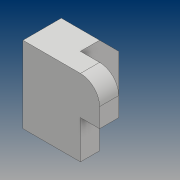
# Autodesk Inventor part: 47 (28785.398 mm^3)
Saved by Autodesk Inventor 2018 (Build 220112000, 112)
## iProperties
Created: 2020-09-18
Part Number: 47 (28785.398 mm^3)
Material: 一般
Document SubType Name: Modeling
Designer: 88697
Density: 1 g/cm^3
Appearance: 預設
Author: 88697
Autodesk Inventor part; units mm, degrees
ref_plane "YZ Plane" through (0, 0, 0) normal (1, 0, 0) x (0, 1, 0)
ref_plane "XZ Plane" through (0, 0, 0) normal (0, 1, 0) x (-1, 0, 0)
ref_plane "XY Plane" through (0, 0, 0) normal (0, 0, 1) x (1, 0, 0)
sketch "草圖1" plane through (0, 0, 0) normal (0, 1, 0) x (-1, 0, 0)
  line L0 (0, 0) -> (-40, 0)
  line L1 (-40, 0) -> (-40, -20)
  line L2 (-30, -40) -> (0, -40)
  line L3 (0, -40) -> (0, 0)
  line L4 (-40, -20) -> (-30, -20)
  line L5 (-30, -20) -> (-30, -40)
  dimension "d0" = 20
  dimension "d1" = 40
  dimension "d2" = 10
  dimension "d3" = 40
  constraints: 12 end point, 2 horizontal, 2 parallel, 1 perpendicular, 1 vertical
  measures "d0" distance of L0.end L1.end
  measures "d1" distance between parallel lines of L0 L2
  measures "d2" distance of L1.end L4.end
  measures "d3" distance of L0.start L0.end
extrude "擠出1" add sketch "草圖1" along normal blind 10
sketch "草圖2" plane through (0, 0, -40) normal (-1, 0, 0) x (0, 0, 1)
  line L0 (20, 10) -> (0, 10) projected
  line L1 (0, 10) -> (40, 10)
  line L2 (40, 10) -> (40, 20)
  line L3 (30, 30) -> (0, 30)
  line L4 (0, 30) -> (0, 10)
  line L5 (40, 20) -> (30, 30)
  line L6 (40, 0) -> (40, 10) projected
  line L7 (0, 0) -> (40, 0) projected
  dimension "d6" = 0
  dimension "d7" = 10
  dimension "d8" = 30
  dimension "d9" = 10
  constraints: 10 end point, 2 parallel, 1 horizontal, 1 perpendicular
  measures "d6" distance between parallel lines of L6 L2
  measures "d7" distance from line of L2.end L3
  measures "d8" distance between parallel lines of L7 L3
  measures "d9" distance from line of L2 L3.start
extrude "擠出2" add sketch "草圖2" against normal blind 20
fillet "圓角1" radius 10 1 edges at (40, 5, 0)
